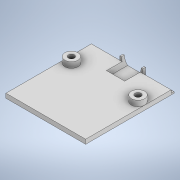
# Autodesk Inventor part: ExpansionCard_SelfTapping_Lid
Saved by Autodesk Inventor 2022 (Build 260153000, 153)
## iProperties
Created: 2022-05-23
Part Number: ExpansionCard_SelfTapping_Lid
Material: Generic
Document SubType Name: Modeling
Designer: SHOP-Station5
Density: 1 g/cm^3
Appearance: Default
Author: SHOP-Station5
Autodesk Inventor part; units mm, degrees
ref_plane "YZ Plane" through (0, 0, 0) normal (1, 0, 0) x (0, 1, 0)
ref_plane "XZ Plane" through (0, 0, 0) normal (0, 1, 0) x (-1, 0, 0)
ref_plane "XY Plane" through (0, 0, 0) normal (0, 0, 1) x (1, 0, 0)
sketch "Sketch1" plane through (0, 0, 0) normal (0, 1, 0) x (-1, 0, 0)
  line L0 (-27.0524, -30.5) -> (0, -30.5)
  line L1 (-27.0524, -30.5) -> (-27.0524, 0)
  line L2 (-27.0524, 0) -> (0, 0)
  line L3 (0, 0) -> (0, -30.5)
  point P0 (-13.5262, -30.5)
  constraints: 8 end point, 1 vertical
extrude "Extrusion1" add sketch "Sketch1" along normal blind 1.5
sketch "Sketch2" plane through (0, 0, 0) normal (0, -1, 0) x (1, 0, 0)
  circle A0 centre (2.2262, -20) radius 2.2262
  circle A1 centre (24.8262, -20) radius 2.2262
  point P0 (0, 0)
  point P1 (13.5262, -30.5)
  point P2 (27.0524, -30.5)
  constraints: 2 centre point
extrude "Extrusion2" add sketch "Sketch2" against normal blind 3.4
sketch "Sketch3" plane through (0, 0, 0) normal (0, -1, 0) x (1, 0, 0)
  circle A0 centre (24.8262, -19.9938) radius 1.016
  circle A1 centre (2.2262, -20) radius 1.016
  point P0 (0, 0)
  point P1 (13.5262, 0)
  point P2 (1.4262, -20)
  point P3 (0, -30.5)
  dimension "d4" = 2.032
  constraints: 2 centre point
  measures "d4" diameter of A0
extrude "Extrusion3" cut sketch "Sketch3" against normal up to surface (3.4 mm away)
sketch "Sketch4" plane through (0, 0, 0) normal (0, -1, 0) x (1, 0, 0)
  circle A0 centre (24.8262, -19.9938) radius 2.032
  circle A1 centre (2.2262, -20) radius 2.032
  line L0 (2.2262, -20) -> (0, -20)
  line L1 (0, -20) -> (0, -30.5)
  line L2 (0, -30.5) -> (0, 0) projected
  point P0 (13.5262, 0)
  dimension "d7" = 4.064
  dimension "d8" = 4.064
  constraints: 4 end point, 2 centre point, 1 coincident, 1 horizontal
  measures "d7" diameter of A0
  measures "d8" diameter of A1
extrude "Extrusion4" cut sketch "Sketch4" against normal blind 2.051
sketch "Sketch8" plane through (0, 0, -30.5) normal (-1, 0, 0) x (0, 0, 1)
  line L0 (0, 0) -> (30.5, 0) projected
  line L1 (0, 0) -> (0, 1.5) projected
  line L2 (0, 0) -> (0, 1.5)
  line L3 (0, 0) -> (0.5, 0)
  line L4 (0.5, 0) -> (0.5, 0.5)
  line L5 (0.5, 0.5) -> (1.5, 0.5)
  line L6 (1.5, 0.5) -> (1.5, 1.5)
  line L7 (0, 1.5) -> (10.5, 1.5) projected
  line L8 (0, 1.5) -> (1.5, 1.5)
  dimension "d23" = 0.5
  dimension "d24" = 0.5
  dimension "d25" = 1
  constraints: 12 end point, 4 perpendicular, 2 point on line, 1 vertical
  measures "d23" distance of L0.start L3.end
  measures "d24" distance of L3.end L4.end
  measures "d25" distance of L4.end L5.end
extrude "Extrusion7" cut sketch "Sketch8" against normal up to surface (27.0524 mm away)
sketch "Sketch9" plane through (27.0524, 0, -30) normal (0, 0, -1) x (-1, 0, 0)
  line L0 (27.0524, 0) -> (0, 0) projected
  line L1 (27.0524, 0.5) -> (27.0524, 0) projected
  line L2 (0, 0) -> (0, 1.5) projected
  line L3 (13.5262, 0) -> (16.8762, 0)
  line L4 (13.5262, 0) -> (10.1762, 0)
  line L5 (13.5262, 2.8) -> (13.5262, 0.3)
  line L6 (13.5262, 0.3) -> (15.7561, 0.3)
  line L7 (13.5262, 0.3) -> (11.2963, 0.3)
  arc A0 (15.7561, 0.3) -> (16.8762, 2.8) centre (13.5262, 2.8) ccw
  arc A1 (10.1762, 2.8) -> (11.2963, 0.3) centre (13.5262, 2.8) ccw
  line L8 (10.1762, 0) -> (9.6762, 0)
  line L9 (9.6762, 0) -> (9.6762, 2.8)
  line L10 (9.6762, 2.8) -> (10.1762, 2.8)
  line L11 (16.8762, 0) -> (17.3762, 0)
  line L12 (17.3762, 0) -> (17.3762, 2.8)
  line L13 (17.3762, 2.8) -> (16.8762, 2.8)
  point P0 (0, 0.5)
  dimension "d29" = 3.35
  dimension "d30" = 3.35
  dimension "d31" = 2.5
  dimension "d32" = 0.5
  dimension "d33" = 0.5
  constraints: 22 end point, 5 point on line, 4 perpendicular, 4 point on circle, 2 centre point, 1 horizontal, 1 midpoint
  measures "d29" distance of L3.start L3.end
  measures "d30" distance of L3.start L4.end
  measures "d31" distance of L5.start L5.end
  measures "d32" distance of L4.end L8.end
  measures "d33" distance of L3.end L11.end
sketch "Sketch10" plane through (27.0524, 0, -30) normal (0, 0, -1) x (-1, 0, 0)
  line L0 (0, 0) -> (0, 1.5) projected
  line L1 (13.5262, 0.25) -> (16.3262, 0.25) construction
  line L2 (13.5262, 0.5) -> (15.8262, 0.5) construction
  line L3 (13.5262, 0.3) -> (11.2963, 0.3)
  line L4 (13.5262, 0.3) -> (15.7561, 0.3)
  arc A0 (15.6987, 0.25) -> (15.9619, 0.5) centre (13.5262, 2.8) ccw
  arc A1 (11.0905, 0.5) -> (11.2963, 0.3) centre (13.5262, 2.8) ccw
  line L5 (0, 1.5) -> (27.0524, 1.5) projected
  line L6 (10.4387, 1.5) -> (16.6137, 1.5)
  arc A2 (15.6987, 0.25) -> (16.6137, 1.5) centre (13.5262, 2.8) ccw
  arc A3 (10.4387, 1.5) -> (11.2963, 0.3) centre (13.5262, 2.8) ccw
  point P0 (0, 0.5)
  dimension "d42" = 0.2
  constraints: 10 end point, 10 point on circle, 4 centre point, 4 point on line, 2 horizontal, 1 coincident
  measures "d42" distance of L2.start L3.start
extrude "Extrusion8" add sketch "Sketch9" against normal up to surface (1 mm away)
extrude "Extrusion9" cut sketch "Sketch10" against normal blind 6.3
body "Solid1"
